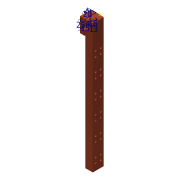
# Autodesk Inventor part: 17-0028-0025
Saved by Autodesk Inventor 2016 SP2 (Build 200236200, 236)
## iProperties
Category: IOP
Company: Universiteit van Amsterdam
Created: 2017-11-02
Part Number: 17-0028-0025
Material: Copper
Document SubType Name: Modeling
Designer: Daan Giesen
Density: 8.94 g/cm^3
Appearance: Copper - Satin
Mass: 1877.4 g
Surface Area: 362 cm^2
Volume: 210 cm^3
Project: Digital PID Loop
Cost Center: 17-0028
User Status: Work in Progress
Authority: Reichsöllner, Lukas
Author: Daan Giesen
Title: Digital PID Loop
Revision Number: A
Autodesk Inventor part; units mm, degrees
ref_plane "YZ Plane" through (0, 0, 0) normal (1, 0, 0) x (0, 1, 0)
ref_plane "XZ Plane" through (0, 0, 0) normal (0, 1, 0) x (-1, 0, 0)
ref_plane "XY Plane" through (0, 0, 0) normal (0, 0, 1) x (1, 0, 0)
sketch "Sketch1" plane through (0, 0, 0) normal (0, 0, 1) x (1, 0, 0)
  line L0 (0, 21) -> (0, -21) construction
  line L1 (-14, 0) -> (14, 0) construction
  line L2 (10, -15) -> (-10, -15)
  line L3 (-10, -15) -> (-10, 15)
  line L4 (-10, 15) -> (10, 15)
  line L5 (10, 15) -> (10, -15)
  line L6 (10, -15) -> (-10, 15) construction
  line L7 (-10, -15) -> (10, 15) construction
  point P0 (0, 0)
  dimension "d4" = 30
  dimension "d5" = 20
  constraints: 12 end point, 2 midpoint, 2 parallel, 1 horizontal, 1 perpendicular
  measures "d4" distance of L4.end L2.start
  measures "d5" distance between parallel lines of L3 L5
extrude "Extrusion3" add sketch "Sketch1" against normal blind 350
sketch "Sketch3" plane through (10, -15, 0) normal (1, 0, 0) x (0, 0, -1)
  circle A0 centre (82.1, 22) radius 2.65 projected
  circle A1 centre (68.1, 8) radius 2.65 projected
  circle A2 centre (82.1, 8) radius 2.65 projected
  circle A3 centre (68.1, 22) radius 2.65 projected
  line L0 (90.1, 40) -> (90.1, 0) projected
  line L1 (60.1, 40) -> (90.1, 40) projected
  line L2 (60.1, 40) -> (60.1, 0) projected
  line L3 (60.1, 0) -> (90.1, 0) projected
  point P0 (0, 15)
extrude "Extrusion4" cut sketch "Sketch3" against normal through all contours A0 | A1 | A2 | A3
pattern_linear "Rectangular Pattern1" count 6 spacing 50 along (0, 0, -1) of "Extrusion4"
sketch "Sketch4" plane through (-10, 15, 0) normal (0, 1, 0) x (1, 0, 0)
  circle A0 centre (-1, 20) radius 7.5
  line L0 (-15, 40) -> (-2, 40)
  line L1 (-2, 0) -> (-15, 0)
  line L2 (-15, 0) -> (-15, 40)
  line L3 (0, 0) -> (0, 350) projected
  line L4 (-2, 40) -> (-2, 27.433)
  line L5 (-2, 12.567) -> (-2, 0)
  point P0 (10, 0)
  dimension "d20" = 15
  dimension "d23" = 13
  dimension "d24" = 40
  dimension "d25" = 20
  constraints: 10 end point, 3 parallel, 2 perpendicular, 2 point on circle, 1 centre point, 1 horizontal, 1 horizontal alignment
  measures "d20" diameter of A0
  measures "d23" distance of L0.start L0.end
  measures "d24" distance of L1.end L0.start
  measures "d25" vertical distance of point (10, 0) A0.centre
extrude "Extrusion5" cut sketch "Sketch4" against normal through all contours A0 L3 | A0 L3
extrude "Extrusion6" add sketch "Sketch4" against normal up to surface (30 mm away) separate body contours A0 L5 L1 L2 L0 L4
sketch "Sketch5" plane through (-25, 15, -40) normal (-1, 0, 0) x (0, 0, 1)
  line L0 (32.5, -7.5) -> (7.5, -7.5) construction
  line L1 (7.5, -7.5) -> (7.5, -22.5) construction
  line L2 (7.5, -22.5) -> (32.5, -22.5) construction
  line L3 (32.5, -22.5) -> (32.5, -7.5) construction
  line L4 (32.5, -7.5) -> (7.5, -22.5) construction
  line L5 (7.5, -7.5) -> (32.5, -22.5) construction
  line L6 (0, 0) -> (40, 0) construction
  line L7 (40, 0) -> (40, -30) construction
  point P0 (40, -15)
  point P1 (20, -15)
  point P2 (20, 0)
  point P3 (20, -15)
  point P4 (20, -15)
  point P5 (40, -15)
  dimension "d30" = 15
  dimension "d31" = 25
  constraints: 12 end point, 6 midpoint, 4 coincident, 2 parallel, 1 horizontal, 1 horizontal alignment, 1 perpendicular, 1 vertical alignment
  measures "d30" distance of L0.end L1.end
  measures "d31" distance of L1.end L2.end
equation "\"d22\" = 0.5 * d21"
equation "\"d21\" = 2"
body "Solid3"
body "Solid4"
